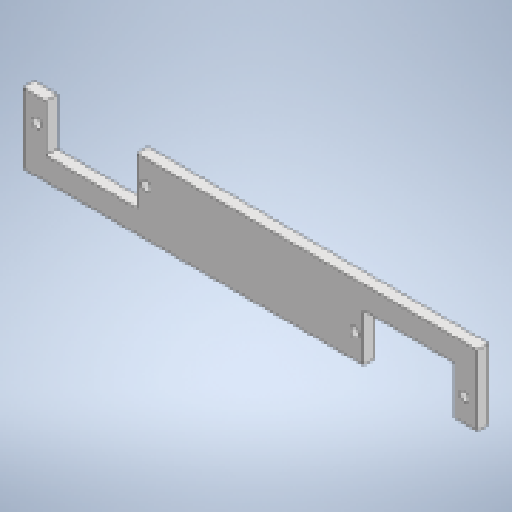
# Autodesk Inventor part: Arm_1
Saved by Autodesk Inventor 2023 (Build 270158000, 158)
## iProperties
Created: 2022-04-08
Part Number: Arm_1
Material: 一般
Document SubType Name: Modeling
Designer: device
Mass: 4.8011 g
Surface Area: 42.7598 cm^2
Volume: 4.8011 cm^3
Density: 1 g/cm^3
Appearance: 預設
Author: device
Autodesk Inventor part; units mm, degrees
ref_plane "YZ Plane" through (0, 0, 0) normal (1, 0, 0) x (0, 1, 0)
ref_plane "XZ Plane" through (0, 0, 0) normal (0, 1, 0) x (-1, 0, 0)
ref_plane "XY Plane" through (0, 0, 0) normal (0, 0, 1) x (1, 0, 0)
sketch "草圖1" plane through (0, 0, 0) normal (0, 0, 1) x (1, 0, 0)
  line L0 (-12, -6.25) -> (12, -6.25)
  line L1 (12, -6.25) -> (12, 6.25)
  line L2 (12, 6.25) -> (-12, 6.25)
  line L3 (-12, 6.25) -> (-12, -6.25)
  line L4 (-12, -6.25) -> (12, 6.25) construction
  line L5 (12, -6.25) -> (-12, 6.25) construction
  line L6 (18, -6.25) -> (-72, -6.25)
  line L7 (-72, -6.25) -> (-72, 12.25)
  line L8 (-72, 12.25) -> (18, 12.25)
  line L9 (18, 12.25) -> (18, -6.25)
  line L10 (-66, 12.25) -> (-42, 12.25)
  line L11 (-42, 12.25) -> (-42, -0.25)
  line L12 (-42, -0.25) -> (-66, -0.25)
  line L13 (-66, -0.25) -> (-66, 12.25)
  point P0 (0, 0)
  point P1 (-66, 6)
  point P2 (12, -6.25)
  point P3 (-42, 12.25)
  dimension "d0" = 24
  dimension "d1" = 12.5
  dimension "d2" = 6
  dimension "d3" = 6
  dimension "d4" = 6
  dimension "d5" = 90
  constraints: 28 end point, 8 parallel, 3 horizontal, 3 midpoint, 3 perpendicular, 1 collinear, 1 point on line
  measures "d0" distance of L1.end L2.end
  measures "d1" distance of L0.end L1.end
  measures "d2" distance between parallel lines of L1 L9
  measures "d3" distance between parallel lines of L2 L8
  measures "d4" distance from line of L7 point (-66, 6)
  measures "d5" distance of L6.start L6.end
extrude "擠出1" add sketch "草圖1" along normal mid plane 3 contours L6 L7 L8 L13 L12 L11 L9 L1 L2 L3
sketch "草圖2" plane through (0, 0, 1.5) normal (0, 0, 1) x (1, 0, 0)
  line L0 (12, 6.25) -> (12, -6.25) construction
  line L1 (12, -6.25) -> (18, -6.25) construction
  line L2 (18, -6.25) -> (18, 12.25) construction
  line L3 (18, 12.25) -> (-42, 12.25) construction
  line L4 (-42, 12.25) -> (-42, -0.25) construction
  line L5 (-42, -0.25) -> (-66, -0.25) construction
  line L6 (-66, -0.25) -> (-66, 12.25) construction
  line L7 (-66, 12.25) -> (-72, 12.25) construction
  line L8 (-72, 12.25) -> (-72, -6.25) construction
  line L9 (-72, -6.25) -> (-12, -6.25) construction
  line L10 (-12, -6.25) -> (-12, 6.25) construction
  line L11 (-12, 6.25) -> (12, 6.25) construction
  line L12 (-14.5, 0) -> (14.5, 0) construction
  circle A0 centre (14.5, 0) radius 1.25
  circle A1 centre (-14.5, 0) radius 1.25
  line L13 (-72, 12.25) -> (18, -6.25) construction
  circle A2 centre (-39.5, 6) radius 1.25
  circle A3 centre (-68.5, 6) radius 1.25
  point P0 (0, 0)
  point P1 (-27, 3)
  dimension "d8" = 2.5
  dimension "d9" = 29
  dimension "d12" = 360
  constraints: 5 end point, 4 centre point, 3 midpoint, 1 coincident, 1 equal radius, 1 horizontal, 9 other
  measures "d8" diameter of A0
  measures "d9" distance of L12.start L12.end
extrude "擠出2" cut sketch "草圖2" against normal up to surface (3 mm away)
equation "\"d4\" = d2"
equation "\"d6\" = w"
equation "\"w\" = 3"
